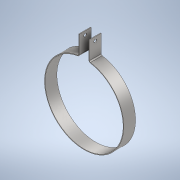
# Autodesk Inventor part: Banda de montaje
Saved by Autodesk Inventor 2021 (Build 250183000, 183)
## iProperties
Created: 2021-07-11
Part Number: Banda de montaje
Material: Generic
Document SubType Name: Modeling
Designer: Nelson
Density: 1 g/cm^3
Appearance: Stainless - Brushed
Author: Nelson
Autodesk Inventor part; units mm, degrees
ref_plane "YZ Plane" through (0, 0, 0) normal (1, 0, 0) x (0, 1, 0)
ref_plane "XZ Plane" through (0, 0, 0) normal (0, 1, 0) x (-1, 0, 0)
ref_plane "XY Plane" through (0, 0, 0) normal (0, 0, 1) x (1, 0, 0)
sketch "Sketch1" plane through (0, 0, 0) normal (0, 0, 1) x (1, 0, 0)
  line L0 (0, 0) -> (0, 19.8871) construction
  arc A0 (-8.0952, 49.3403) -> (8.0952, 49.3403) centre (0, 0) ccw
  arc A1 (-8.241, 50.2284) -> (8.241, 50.2284) centre (0, 0) ccw
  line L1 (-6, 74.4853) -> (-6, 51.8073)
  arc A2 (-8.0952, 49.3403) -> (-6, 51.8073) centre (-8.5, 51.8073) ccw
  arc A3 (-8.241, 50.2284) -> (-6.9, 51.8073) centre (-8.5, 51.8073) ccw
  line L2 (-6.9, 51.8073) -> (-6.9, 74.4853)
  line L3 (-6.9, 74.4853) -> (-6, 74.4853)
  line L4 (6, 74.4853) -> (6, 51.8073)
  arc A4 (6, 51.8073) -> (8.0952, 49.3403) centre (8.5, 51.8073) ccw
  arc A5 (6.9, 51.8073) -> (8.241, 50.2284) centre (8.5, 51.8073) ccw
  line L5 (6.9, 51.8073) -> (6.9, 74.4853)
  line L6 (6.9, 74.4853) -> (6, 74.4853)
  point P0 (-6.455, 50.3692)
  point P1 (6.455, 50.3692)
  dimension "d32" = 5
  dimension "d33" = 6
  dimension "d34" = 0.9
  dimension "d44" = 50
  dimension "d45" = 50.9
  dimension "d46" = 22.678
  constraints: 14 end point, 14 point on circle, 8 symmetric about line, 6 centre point, 2 coincident, 2 tangent, 2 vertical, 1 horizontal, 3 other
  measures "d32" diameter of A2
  measures "d33" distance from line of L0.start L1
  measures "d34" radial gap between concentric circles of A2 A3
  measures "d44" radius of A0
  measures "d45" radius of A1
  measures "d46" distance of L2.start L2.end
extrude "Extrusion1" add sketch "Sketch1" against normal blind 15
sketch "Sketch2" plane through (-6.9, 51.8073, 0) normal (-1, 0, 0) x (0, 0, 1)
  line L0 (0, 22.678) -> (-15, 22.678) projected
  line L1 (0, 22.678) -> (0, 0) projected
  point P0 (0, -51.8073)
  point P1 (-7.5, 17.878)
  dimension "d35" = 4.8
  dimension "d43" = 7.5
  measures "d35" distance from line of L0 point (-7.5, 17.878)
  measures "d43" distance from line of L1 point (-7.5, 17.878)
hole "Hole1" at (-6.9, 69.6853, -7.5) direction (1, 0, 0) diameter 4 depth 25 tip angle 137
body "Solid1"
